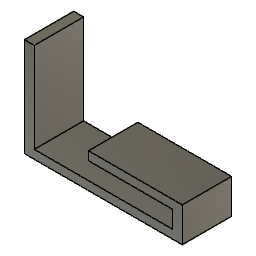
bracket v3 (Autodesk Fusion 360 design; units mm, degrees)
Autodesk Fusion 360 part; units mm, degrees
sketch "Sketch1" plane through (0, 0, 0) normal (0, 1, 0) x (1, 0, 0)
  line L0 (0, 0) -> (28, 0)
  line L1 (28, 0) -> (28, -7)
  line L2 (28, -7) -> (13, -7)
  line L3 (13, -7) -> (13, -5)
  line L4 (13, -5) -> (26, -5)
  line L5 (26, -5) -> (26, -2)
  line L6 (26, -2) -> (2, -2)
  line L7 (2, -2) -> (2, -20)
  line L8 (2, -20) -> (0, -20)
  line L9 (0, -20) -> (0, 0)
  constraint coincident L0.start L9.end
  constraint horizontal L0
  constraint perpendicular L0 L1
  constraint perpendicular L1 L2
  constraint perpendicular L2 L3
  constraint perpendicular L3 L4
  constraint perpendicular L4 L5
  constraint perpendicular L5 L6
  constraint perpendicular L6 L7
  constraint perpendicular L7 L8
  constraint perpendicular L0 L9
extrude "Extrude1" add sketch "Sketch1" along normal blind 10
extrude "Extrude2" add 1 faces at (28, 3.3333, 2.3333) along direction (1, 0, 0) blind 4
extrude "Extrude3" cut 1 faces at (26, 3.3333, 4) along direction (1, 0, 0) blind 4
extrude "Extrude4" cut 1 faces at (18.6667, 3.3333, 5) along direction (0, 0, 1) blind 0.25
extrude "Extrude5" cut 1 faces at (11.3333, 3.3333, 2) along direction (0, 0, -1) blind 0.25
